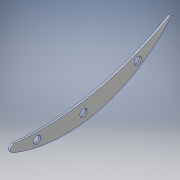
# Autodesk Inventor part: element_base
Saved by Autodesk Inventor 2018.1 (Build 221171000, 171)
## iProperties
Created: 2017-10-22
Part Number: element_base
Material: アルミニウム 6061
Document SubType Name: Modeling
Designer: ku_sk
Mass: 222.517 g
Surface Area: 387.371 cm^2
Volume: 82.4138 cm^3
Density: 2.7 g/cm^3
Appearance: アルミニウム - フラット
Author: ku_sk
Autodesk Inventor part; units mm, degrees
ref_plane "YZ Plane" through (0, 0, 0) normal (1, 0, 0) x (0, 1, 0)
ref_plane "XZ Plane" through (0, 0, 0) normal (0, 1, 0) x (-1, 0, 0)
ref_plane "XY Plane" through (0, 0, 0) normal (0, 0, 1) x (1, 0, 0)
sketch "スケッチ1" plane through (0, 0, 0) normal (1, 0, 0) x (0, 1, 0)
  line L0 (0, 250) -> (88.1635, -250)
  arc A0 (0, 250) -> (88.1635, -250) centre (710.7652, 117.5543) ccw
  arc A1 (0, 250) -> (88.1635, -250) centre (325.1936, 49.5676) ccw
  line L1 (0, -370.1192) -> (0, 353.3532) projected
  point P0 (0, 0)
  dimension "d0" = 250
  dimension "d2" = 500
  dimension "d3" = 10
  dimension "d4" = 723
  dimension "d5" = 382
  constraints: 4 point on circle, 2 centre point, 2 end point, 1 point on line
  measures "d0" distance of L0.start point (0, 0)
  measures "d2" vertical distance of L0.start L0.end
  measures "d3" angle of L1 L0
  measures "d4" radius of A0
  measures "d5" radius of A1
extrude "押し出し1" add sketch "スケッチ1" along normal mid plane 5 contours A0 L1 A1 | A1 L1 A0
sketch "スケッチ3" plane through (0, 0, 0) normal (1, 0, 0) x (0, 1, 0)
  circle A0 centre (-30, 128) radius 10
  circle A1 centre (-30, 0) radius 10
  circle A2 centre (20, -150) radius 10
  line L0 (-54, 0) -> (44, 0) projected
  line L1 (0, -219.6) -> (0, 197.6) projected
  point P0 (0, 0)
  dimension "d10" = 128
  dimension "d11" = 30
  dimension "d12" = 20
  dimension "d13" = 20
  dimension "d14" = 20
  dimension "d15" = 30
  dimension "d16" = 150
  dimension "d19" = 20
  constraints: 3 centre point, 1 point on line
  measures "d10" vertical distance of point (0, 0) A0.centre
  measures "d11" horizontal distance of A0.centre point (0, 0)
  measures "d12" diameter of A0
  measures "d13" diameter of A1
  measures "d14" diameter of A2
  measures "d15" distance of point (0, 0) A1.centre
  measures "d16" distance from line of L0 A2.centre
  measures "d19" distance from line of L1 A2.centre
extrude "押し出し2" cut sketch "スケッチ3" along normal through all both and the other way through all
fillet "フィレット1" radius 10 1 edges at (0, 0, 250)
fillet "フィレット2" radius 2 1 edges at (0, 88.1635, -250)
